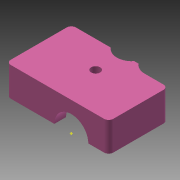
# Autodesk Inventor part: hotend-holder-front
Saved by Autodesk Inventor 2014 (Build 180170000, 170)
## iProperties
Created: 2013-12-31
Part Number: hotend-holder-front
Material: Generic
Document SubType Name: Modeling
Designer: caleb
Density: 1 g/cm^3
Appearance: Pink
Author: caleb
Autodesk Inventor part; units mm, degrees
ref_plane "YZ Plane" through (0, 0, 0) normal (1, 0, 0) x (0, 1, 0)
ref_plane "XZ Plane" through (0, 0, 0) normal (0, 1, 0) x (-1, 0, 0)
sketch "Sketch1" plane through (0, 0, 0) normal (0, 0, 1) x (1, 0, 0)
  line L0 (0, 0) -> (36.2, 0)
  line L1 (36.2, 0) -> (36.2, 23)
  line L2 (36.2, 23) -> (0, 23)
  line L3 (0, 23) -> (0, 0)
  dimension "d0" = 36.2
  dimension "d1" = 23
  constraints: 8 end point, 2 parallel, 1 horizontal, 1 perpendicular
  measures "d0" distance of L0.start L0.end
  measures "d1" distance of L2.end L0.start
extrude "Extrusion1" add sketch "Sketch1" against normal blind 10.32
sketch "Sketch2" plane through (0, 0, 0) normal (0, 0, 1) x (1, 0, 0)
  line L0 (0, 0) -> (36.2, 0) projected
  line L1 (36.2, 0) -> (36.2, 23) projected
  circle A0 centre (18.1, 13.5) radius 1.5
  dimension "d4" = 3
  dimension "d5" = 18.1
  dimension "d6" = 13.5
  constraints: 1 centre point, 1 coincident
  measures "d4" diameter of A0
  measures "d5" distance from line of L1 A0.centre
  measures "d6" distance from line of L0 A0.centre
hole "Hole1" at (18.1, 13.5, 0) direction (0, 0, -1) diameter 3.2 end through all clearance for "Flat Head Machine Screw" size "M3" standard "Ansi Metric M Profile"
sketch "Sketch3" plane through (0, 0, 0) normal (0, 0, 1) x (1, 0, 0)
  circle A0 centre (18.1, 13.5) radius 1.6 projected
  line L0 (0, 0) -> (36.2, 0) projected
  line L1 (36.2, 0) -> (36.2, 23) projected
  line L2 (36.2, 23) -> (0, 23) projected
  line L3 (0, 23) -> (0, 0) projected
  line L4 (36.2, 21) -> (27.9042, 21)
  arc A1 (23.7521, 23) -> (27.9042, 21) centre (27.9042, 26.31) ccw
  arc A2 (13.9479, 23) -> (22.2521, 23) centre (18.1, 26.31) ccw
  line L5 (18.1, 21) -> (18.1, 0) construction
  dimension "d14" = 3.2
  dimension "d15" = 21
  dimension "d16" = 5.31
  dimension "d17" = 1.5
  constraints: 5 point on circle, 4 end point, 4 point on line, 2 centre point, 1 equal radius, 1 horizontal alignment, 1 midpoint, 1 perpendicular, 1 tangent, 1 vertical alignment
  measures "d14" diameter of A0
  measures "d15" distance between parallel lines of L0 L4
  measures "d16" radius of A2
  measures "d17" distance of A2.end A1.start
extrude "Extrusion2" cut sketch "Sketch3" against normal blind 10.32 contours L4 A1 L2 L1 | L2 A2
sketch "Sketch4" plane through (0, 0, -10.32) normal (0, 0, -1) x (-1, 0, 0)
  circle A0 centre (-18.1, 13.5) radius 1.6 projected
  line L0 (-36.2, 21) -> (-36.2, 0) projected
  line L1 (0, 0) -> (0, 23) projected
  circle A1 centre (-31.1, 13.5) radius 3
  circle A2 centre (-5.1, 13.5) radius 3
  line L2 (-34.1, 13.5) -> (-36.2, 13.5)
  line L3 (-2.1, 13.5) -> (0, 13.5)
  point P0 (-35.15, 13.5)
  dimension "d21" = 6
  dimension "d20" = 26
  constraints: 5 horizontal alignment, 4 end point, 2 collinear, 2 perpendicular, 2 point on line, 1 midpoint, 4 other
  measures "d20" distance of point (-5.1, 13.5) point (-31.1, 13.5)
extrude "Extrusion3" cut sketch "Sketch4" against normal blind 4.7 contours A1 | A2
sketch "Sketch6" plane through (0, 0, -10.32) normal (0, 0, -1) x (-1, 0, 0)
  line L0 (-22.2521, 23) -> (-23.7521, 23) projected
  line L1 (-36.2, 0) -> (0, 0) projected
  line L2 (-33.0021, 4.13) -> (-13.0021, 4.13)
  line L3 (-13.0021, 4.13) -> (-13.0021, 9.88)
  line L4 (-13.0021, 9.88) -> (-33.0021, 9.88)
  line L5 (-33.0021, 9.88) -> (-33.0021, 4.13)
  point P0 (-23.0021, 23)
  point P1 (-23.0021, 9.88)
  dimension "d27" = 5.75
  dimension "d28" = 20
  dimension "d29" = 4.13
  constraints: 8 end point, 2 midpoint, 2 parallel, 1 horizontal, 1 perpendicular, 1 vertical alignment
  measures "d27" distance of L2.end L3.end
  measures "d28" distance of L2.start L2.end
  measures "d29" distance between parallel lines of L1 L2
extrude "Extrusion5" cut sketch "Sketch6" against normal blind 8.73
fillet "Fillet1" radius 1.5875 4 edges at (13.0021, 9.88, -5.955) (13.0021, 4.13, -5.955) (33.0021, 9.88, -5.955) (33.0021, 4.13, -5.955)
fillet "Fillet2" radius 1.5875 4 edges at (36.2, 21, -5.16) (36.2, 0, -5.16) (0, 0, -5.16) (0, 23, -5.16)
sketch "Sketch5" plane through (0, 0, 0) normal (0, -1, 0) x (1, 0, 0)
  line L0 (23.7521, 0) -> (22.2521, 0) projected
  circle A0 centre (23.0021, 0) radius 1 construction
  line L1 (36.2, -10.32) -> (0, -10.32) projected
  circle A1 centre (23.0021, -10.32) radius 1
  dimension "d24" = 2
  constraints: 2 centre point, 1 equal radius, 1 midpoint, 1 point on line, 1 vertical alignment
  measures "d24" diameter of A0
extrude "Extrusion4" cut sketch "Sketch5" against normal through all
sketch "Sketch7" plane through (1.5875, 0, 0) normal (0, -1, 0) x (1, 0, 0)
  arc A0 (22.4146, -10.32) -> (20.4146, -10.32) centre (21.4146, -10.32) ccw projected
  circle A1 centre (21.4146, -10.32) radius 6
  point P0 (-1.5875, 0)
  dimension "d34" = 12
  constraints: 1 centre point, 1 coincident
  measures "d34" diameter of A1
extrude "Extrusion6" cut sketch "Sketch7" against normal up to surface (4.13 mm away)
ref_plane "Work Plane1" through (23.0021, 0, -10.32) normal (1, 0, 0) x (0, 0, -1)
body "Solid1"
